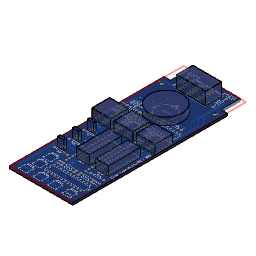
v2 - Timer - PCB (Autodesk Fusion 360 design; units mm, degrees)
Autodesk Fusion 360 part; units mm, degrees
sketch "Sketch1" plane through (0, 0, 0) normal (0, 0, 1) x (1, 0, 0)
  line L0 (0, 0) -> (50, 0)
  line L1 (50, 0) -> (50, 137)
  line L2 (50, 137) -> (0, 137)
  line L3 (0, 137) -> (0, 0)
  line L4 (6, 57.4) -> (11, 57.4)
  line L5 (11, 57.4) -> (11, 55.4)
  line L6 (11, 55.4) -> (6, 55.4)
  line L7 (6, 55.4) -> (6, 57.4)
  line L8 (6, 45.7) -> (11, 45.7)
  line L9 (11, 45.7) -> (11, 43.7)
  line L10 (11, 43.7) -> (6, 43.7)
  line L11 (6, 43.7) -> (6, 45.7)
  line L12 (6, 34) -> (11, 34)
  line L13 (11, 34) -> (11, 32)
  line L14 (11, 32) -> (6, 32)
  line L15 (6, 32) -> (6, 34)
  line L16 (36, 57.4) -> (46.1, 57.4)
  line L17 (46.1, 57.4) -> (46.1, 32)
  line L18 (46.1, 32) -> (36, 32)
  line L19 (36, 32) -> (36, 57.4)
  line L20 (20.9, 57.4) -> (31, 57.4)
  line L21 (31, 57.4) -> (31, 32)
  line L22 (31, 32) -> (20.9, 32)
  line L23 (20.9, 32) -> (20.9, 57.4)
  line L24 (0.1, 79) -> (7.5, 79)
  line L25 (7.5, 79) -> (7.5, 65)
  line L26 (7.5, 65) -> (0.1, 65)
  line L27 (0.1, 65) -> (0.1, 79)
  line L28 (7.5, 65) -> (7.5, 79)
  line L29 (42.5, 79) -> (49.9, 79)
  line L30 (49.9, 79) -> (49.9, 65)
  line L31 (49.9, 65) -> (42.5, 65)
  line L32 (42.5, 65) -> (42.5, 79)
  line L33 (7.5, 79) -> (14.9, 79)
  line L34 (14.9, 79) -> (14.9, 65)
  line L35 (14.9, 65) -> (7.5, 65)
  line L36 (7.5, 65) -> (7.5, 79)
  line L37 (42.5, 79) -> (35.1, 79)
  line L38 (35.1, 79) -> (35.1, 65)
  line L39 (35.1, 65) -> (42.5, 65)
  line L40 (42.5, 65) -> (42.5, 79)
  line L41 (15.25, 79) -> (17.25, 79)
  line L42 (17.25, 79) -> (17.25, 76)
  line L43 (17.25, 76) -> (15.25, 76)
  line L44 (15.25, 76) -> (15.25, 79)
  line L45 (17.6, 79) -> (25, 79)
  line L46 (25, 79) -> (25, 65)
  line L47 (25, 65) -> (17.6, 65)
  line L48 (17.6, 65) -> (17.6, 79)
  line L49 (25, 79) -> (32.4, 79)
  line L50 (32.4, 79) -> (32.4, 65)
  line L51 (32.4, 65) -> (25, 65)
  line L52 (25, 65) -> (25, 79)
  line L53 (32.75, 78.921) -> (34.75, 78.921)
  line L54 (34.75, 78.921) -> (34.75, 75.921)
  line L55 (34.75, 75.921) -> (32.75, 75.921)
  line L56 (32.75, 75.921) -> (32.75, 78.921)
  line L57 (15.25, 68.4103) -> (17.25, 68.4103)
  line L58 (17.25, 68.4103) -> (17.25, 65.4103)
  line L59 (17.25, 65.4103) -> (15.25, 65.4103)
  line L60 (15.25, 65.4103) -> (15.25, 68.4103)
  line L61 (32.75, 68) -> (34.75, 68)
  line L62 (34.75, 68) -> (34.75, 65)
  line L63 (34.75, 65) -> (32.75, 65)
  line L64 (32.75, 65) -> (32.75, 68)
  line L65 (13.6, 131) -> (21.2, 131)
  line L66 (21.2, 131) -> (21.2, 118.3)
  line L67 (21.2, 118.3) -> (13.6, 118.3)
  line L68 (13.6, 118.3) -> (13.6, 131)
  line L69 (21.2, 131) -> (28.8, 131)
  line L70 (28.8, 131) -> (36.4, 131)
  line L71 (36.4, 131) -> (36.4, 118.3)
  line L72 (36.4, 118.3) -> (28.8, 118.3)
  line L73 (28.8, 118.3) -> (28.8, 131)
  line L74 (21.2, 131) -> (28.8, 131)
  line L75 (28.8, 131) -> (28.8, 118.3)
  line L76 (28.8, 118.3) -> (21.2, 118.3)
  line L77 (21.2, 118.3) -> (21.2, 131)
  circle A0 centre (25, 98.3) radius 13
  line L78 (7, 135) -> (12, 135)
  line L79 (12, 135) -> (12, 133)
  line L80 (12, 133) -> (7, 133)
  line L81 (7, 133) -> (7, 135)
  line L82 (38, 135) -> (43, 135)
  line L83 (43, 135) -> (43, 133)
  line L84 (43, 133) -> (38, 133)
  line L85 (38, 133) -> (38, 135)
  line L86 (5, 9) -> (11, 9)
  line L87 (11, 9) -> (11, 3)
  line L88 (11, 3) -> (5, 3)
  line L89 (5, 3) -> (5, 9)
  line L90 (39, 9) -> (45, 9)
  line L91 (45, 9) -> (45, 3)
  line L92 (45, 3) -> (39, 3)
  line L93 (39, 3) -> (39, 9)
  line L94 (16.33, 9) -> (22.33, 9)
  line L95 (22.33, 9) -> (22.33, 3)
  line L96 (22.33, 3) -> (16.33, 3)
  line L97 (16.33, 3) -> (16.33, 9)
  line L98 (27.66, 9) -> (33.66, 9)
  line L99 (33.66, 9) -> (33.66, 3)
  line L100 (33.66, 3) -> (27.66, 3)
  line L101 (27.66, 3) -> (27.66, 9)
  line L102 (7, 26) -> (13, 26)
  line L103 (13, 26) -> (13, 20)
  line L104 (13, 20) -> (7, 20)
  line L105 (7, 20) -> (7, 26)
  line L106 (7, 17.5) -> (13, 17.5)
  line L107 (13, 17.5) -> (13, 11.5)
  line L108 (13, 11.5) -> (7, 11.5)
  line L109 (7, 11.5) -> (7, 17.5)
  circle A1 centre (4, 116) radius 1.5
  circle A2 centre (46, 116) radius 1.5
  line L110 (0, 137) -> (5, 137)
  line L111 (5, 137) -> (5, 122)
  line L112 (5, 122) -> (0, 122)
  line L113 (0, 122) -> (0, 137)
  line L114 (50, 137) -> (45, 137)
  line L115 (45, 137) -> (45, 122)
  line L116 (45, 122) -> (50, 122)
  line L117 (50, 122) -> (50, 137)
  circle A3 centre (25, 98.3) radius 7.5
  dimension "d1" = 50
  dimension "d2" = 137
  dimension "d4" = 2
  dimension "d5" = 6
  dimension "d6" = 5
  dimension "d7" = 2
  dimension "d8" = 6
  dimension "d9" = 5
  dimension "d10" = 2
  dimension "d11" = 6
  dimension "d16" = 32
  dimension "d17" = 10.1
  dimension "d18" = 25.4
  dimension "d19" = 32
  dimension "d20" = 25.4
  dimension "d21" = 9.7
  dimension "d22" = 10.1
  dimension "d23" = 25.4
  dimension "d24" = 32
  dimension "d25" = 5
  dimension "d26" = 7.4
  dimension "d27" = 14
  dimension "d29" = 65
  dimension "d45" = 0.1
  dimension "d47" = 14
  dimension "d48" = 0.1
  dimension "d50" = 14
  dimension "d52" = 14
  dimension "d53" = 65
  dimension "d56" = 2
  dimension "d57" = 3
  dimension "d58" = 0.35
  dimension "d59" = 7.4
  dimension "d60" = 14
  dimension "d61" = 0.35
  dimension "d62" = 7.4
  dimension "d63" = 14
  dimension "d64" = 2
  dimension "d65" = 3
  dimension "d66" = 0.35
  dimension "d67" = 2
  dimension "d68" = 3
  dimension "d69" = 0.35
  dimension "d70" = 2
  dimension "d71" = 3
  dimension "d72" = 0.35
  dimension "d73" = 7.6
  dimension "d74" = 12.7
  dimension "d75" = 7.6
  dimension "d76" = 7.6
  dimension "d77" = 12.7
  dimension "d78" = 6
  dimension "d79" = 13.6
  dimension "d80" = 26
  dimension "d81" = 25
  dimension "d82" = 20
  dimension "d83" = 5
  dimension "d84" = 2
  dimension "d85" = 5
  dimension "d86" = 2
  dimension "d87" = 7
  dimension "d88" = 7
  dimension "d91" = 6
  dimension "d92" = 6
  dimension "d93" = 5
  dimension "d94" = 6
  dimension "d95" = 6
  dimension "d96" = 3
  dimension "d97" = 3
  dimension "d98" = 5
  dimension "d101" = 6
  dimension "d102" = 6
  dimension "d103" = 5.33
  dimension "d104" = 5.33
  dimension "d105" = 6
  dimension "d106" = 6
  dimension "d107" = 6
  dimension "d108" = 6
  dimension "d109" = 2.5
  dimension "d110" = 2.5
  dimension "d111" = 7
  dimension "d112" = 7
  dimension "d113" = 3
  dimension "d114" = 3
  dimension "d115" = 21
  dimension "d116" = 4
  dimension "d117" = 4
  dimension "d118" = 21
  dimension "d133" = 5
  dimension "d134" = 15
  dimension "d135" = 5
  dimension "d136" = 15
  dimension "d151" = 2
  dimension "d152" = 2
  dimension "d153" = 15
  constraint horizontal L0
  constraint vertical L1
  constraint horizontal L2
  constraint vertical L3
  constraint coincident L0.start L3.end
  constraint horizontal L4
  constraint vertical L5
  constraint horizontal L6
  constraint vertical L7
  constraint horizontal L8
  constraint vertical L9
  constraint horizontal L10
  constraint vertical L11
  constraint horizontal L12
  constraint vertical L13
  constraint horizontal L14
  constraint vertical L15
  constraint horizontal L16
  constraint vertical L17
  constraint horizontal L18
  constraint vertical L19
  constraint horizontal L20
  constraint vertical L21
  constraint horizontal L22
  constraint vertical L23
  constraint horizontal L24
  constraint horizontal L26
  constraint vertical L27
  constraint horizontal L29
  constraint vertical L30
  constraint horizontal L31
  constraint vertical L32
  constraint horizontal L33
  constraint vertical L34
  constraint horizontal L35
  constraint vertical L36
  constraint horizontal L37
  constraint vertical L38
  constraint horizontal L39
  constraint vertical L40
  constraint horizontal L41
  constraint vertical L42
  constraint horizontal L43
  constraint vertical L44
  constraint horizontal L45
  constraint vertical L46
  constraint horizontal L47
  constraint vertical L48
  constraint horizontal L49
  constraint vertical L50
  constraint horizontal L51
  constraint vertical L52
  constraint horizontal L53
  constraint vertical L54
  constraint horizontal L55
  constraint vertical L56
  constraint horizontal L57
  constraint vertical L58
  constraint horizontal L59
  constraint vertical L60
  constraint horizontal L61
  constraint vertical L62
  constraint horizontal L63
  constraint vertical L64
  constraint horizontal L65
  constraint vertical L66
  constraint horizontal L67
  constraint vertical L68
  constraint horizontal L69
  constraint horizontal L70
  constraint vertical L71
  constraint horizontal L72
  constraint vertical L73
  constraint horizontal L74
  constraint vertical L75
  constraint horizontal L76
  constraint vertical L77
  constraint horizontal L78
  constraint vertical L79
  constraint horizontal L80
  constraint vertical L81
  constraint horizontal L82
  constraint vertical L83
  constraint horizontal L84
  constraint vertical L85
  constraint horizontal L86
  constraint vertical L87
  constraint horizontal L88
  constraint vertical L89
  constraint horizontal L90
  constraint vertical L91
  constraint horizontal L92
  constraint vertical L93
  constraint horizontal L94
  constraint vertical L95
  constraint horizontal L96
  constraint vertical L97
  constraint horizontal L98
  constraint vertical L99
  constraint horizontal L100
  constraint vertical L101
  constraint horizontal L102
  constraint vertical L103
  constraint horizontal L104
  constraint vertical L105
  constraint horizontal L106
  constraint vertical L107
  constraint horizontal L108
  constraint vertical L109
  constraint horizontal L110
  constraint vertical L111
  constraint horizontal L112
  constraint vertical L113
  constraint horizontal L114
  constraint vertical L115
  constraint horizontal L116
  constraint vertical L117
  constraint concentric A0 A3
  measures "d1" distance of L0.start L0.end
  measures "d2" distance of L0.start L2.end
  measures "d4" distance of L4.start L6.end
  measures "d5" distance of L3 L7
  measures "d6" distance of L8.start L8.end
  measures "d7" distance of L8.start L10.end
  measures "d8" distance of L3 L11
  measures "d9" distance of L12.start L12.end
  measures "d10" distance of L12.start L14.end
  measures "d11" distance of L3 L15
  measures "d16" distance of L0 L14
  measures "d17" distance of L16.start L16.end
  measures "d18" distance of L16.start L18.end
  measures "d19" distance of L0 L18
  measures "d20" distance of L4 L14
  measures "d21" distance of L6 L8
  measures "d22" distance of L20.start L20.end
  measures "d23" distance of L20.start L22.end
  measures "d24" distance of L0 L22
  measures "d25" distance of L19 L21
  measures "d26" distance of L24.start L24.end
  measures "d27" distance of L24.start L26.end
  measures "d29" distance of L0 L26
  measures "d45" distance of L3 L27
  measures "d47" distance of L29.start L31.end
  measures "d48" distance of L1 L30
  measures "d50" distance of L24.end L25.end
  measures "d52" distance of L29.start L31.end
  measures "d53" distance of L0 L31
  measures "d56" distance of L41.start L41.end
  measures "d57" distance of L41.start L43.end
  measures "d58" distance of L34 L44
  measures "d59" distance of L45.start L45.end
  measures "d60" distance of L45.start L47.end
  measures "d61" distance of L42 L48
  measures "d62" distance of L45.end L49.end
  measures "d63" distance of L45.end L46.end
  measures "d64" distance of L53.start L53.end
  measures "d65" distance of L53.start L55.end
  measures "d66" distance of L50 L56
  measures "d67" distance of L57.start L57.end
  measures "d68" distance of L57.start L59.end
  measures "d69" distance of L34 L60
  measures "d70" distance of L61.start L61.end
  measures "d71" distance of L61.start L63.end
  measures "d72" distance of L50 L64
  measures "d73" distance of L65.start L65.end
  measures "d74" distance of L65.start L67.end
  measures "d75" distance of L65.end L69.end
  measures "d76" distance of L69.end L70.end
  measures "d77" distance of L69.end L72.end
  measures "d78" distance of L2 L65
  measures "d79" distance of L3 L68
  measures "d80" diameter of A0
  measures "d81" distance of L3 A0.centre
  measures "d82" distance of L76 A0.centre
  measures "d83" distance of L78.start L78.end
  measures "d84" distance of L78.start L80.end
  measures "d85" distance of L82.start L82.end
  measures "d86" distance of L82.start L84.end
  measures "d87" distance of L3 L81
  measures "d88" distance of L1 L83
  measures "d91" distance of L86.start L86.end
  measures "d92" distance of L86.start L88.end
  measures "d93" distance of L3 L89
  measures "d94" distance of L90.start L90.end
  measures "d95" distance of L90.start L92.end
  measures "d96" distance of L0 L88
  measures "d97" distance of L0 L92
  measures "d98" distance of L1 L91
  measures "d101" distance of L94.start L94.end
  measures "d102" distance of L94.start L96.end
  measures "d103" distance of L87 L97
  measures "d104" distance of L95 L101
  measures "d105" distance of L102.start L102.end
  measures "d106" distance of L102.start L104.end
  measures "d107" distance of L106.start L106.end
  measures "d108" distance of L106.start L108.end
  measures "d109" distance of L104 L106
  measures "d110" distance of L86 L108
  measures "d111" distance of L3 L109
  measures "d112" distance of L3 L105
  measures "d113" diameter of A1
  measures "d114" diameter of A2
  measures "d115" distance of L2 A2.centre
  measures "d116" distance of L1 A2.centre
  measures "d117" distance of L3 A1.centre
  measures "d118" distance of L2 A1.centre
  measures "d133" distance of L2.end L110.end
  measures "d134" distance of L2.end L112.end
  measures "d135" distance of L1.end L114.end
  measures "d136" distance of L1.end L116.end
  measures "d151" distance of L2 L78
  measures "d152" distance of L2 L82
  measures "d153" diameter of A3
extrude "Extrude3" add sketch "Sketch1" against normal blind 1.6 contours L0 L1 L2 L3 L111 L112 L115 L116 | L2 L3 L110 L111 L112 L113 | L1 L2 L114 L115 L116 L117 | L4 L5 L6 L7 | L8 L9 L10 L11 | L12 L13 L14 L15 | L16 L17 L18 L19 | L20 L21 L22 L23 | L24 L25 L26 L27 L28 L36 | L25 L28 L33 L34 L35 L36 | L29 L30 L31 L32 L40 | L32 L37 L38 L39 L40 | L41 L42 L43 L44 | L45 L46 L47 L48 L52 | L46 L49 L50 L51 L52 | L53 L54 L55 L56 | L57 L58 L59 L60 | L61 L62 L63 L64 | L65 L66 L67 L68 L77 | L66 L69 L73 L74 L75 L76 L77 | L70 L71 L72 L73 L75 | A0 | L78 L79 L80 L81 | L82 L83 L84 L85 | L86 L87 L88 L89 | L90 L91 L92 L93 | L94 L95 L96 L97 | L98 L99 L100 L101 | L102 L103 L104 L105 | L106 L107 L108 L109 | A3
extrude "Extrude4" add sketch "Sketch1" along normal blind 7.2 contours L24 L25 L26 L27 L28 L36 | L25 L28 L33 L34 L35 L36 | L29 L30 L31 L32 L40 | L32 L37 L38 L39 L40 | L45 L46 L47 L48 L52 | L46 L49 L50 L51 L52
extrude "Extrude5" add sketch "Sketch1" along normal blind 7 contours L65 L66 L67 L68 L77 | L66 L69 L73 L74 L75 L76 L77 | L70 L71 L72 L73 L75
extrude "Extrude6" add sketch "Sketch1" along normal blind 7.2 contours L16 L17 L18 L19 | L20 L21 L22 L23
extrude "Extrude7" add sketch "Sketch1" along normal blind 7.2 contours L4 L5 L6 L7 | L8 L9 L10 L11 | L12 L13 L14 L15
extrude "Extrude8" cut sketch "Sketch1" against normal blind 15 contours L2 L3 L110 L111 L112 L113 | L1 L2 L114 L115 L116 L117
extrude "Extrude9" add sketch "Sketch1" along normal blind 7.9 contours A0 | A3
extrude "Extrude10" add 1 faces at (21.0958, 100.1802, 7.9) along direction (0, 0, 1) blind 2
extrude "Extrude11" add 1 faces at (21.0958, 100.1802, 9.9) along direction (0, 0, 1) blind 6
extrude "Extrude12" add 1 faces at (28.8, 122.5333, 7) along direction (0, 0, 1) blind 8
extrude "Extrude13" cut 1 faces at (21.0958, 100.1802, 15.9) along direction (0, 0, -1) blind 10
extrude "Extrude14" cut 1 faces at (28.8, 122.5333, 15) along direction (0, 0, -1) blind 5
